BoutonVolume (Autodesk Fusion 360 design; units mm, degrees)
Autodesk Fusion 360 part; units mm, degrees
sketch "Revolution Sketch" plane through (0, 0, 0) normal (0, 1, 0) x (1, 0, 0)
  line L0 (5.5, 0) -> (0, 0)
  line L1 (5.6414, -11.9992) -> (5.5, 0)
  line L2 (-5.8686, 0) -> (0, 0) construction
  line L3 (5.6414, -12) -> (0, -12) construction
  arc A0 (0, -19) -> (12, -15.6532) centre (0.1354, 3.7013) ccw
  line L4 (11.9997, -11.2) -> (12, -13.3255) construction
  line L5 (12, -18.8) -> (12, -15.6532) construction
  line L6 (12, -14.6532) -> (12, -13.3255) construction
  line L7 (12, -18.8) -> (12, -15.6532) construction
  line L8 (12, -14.6532) -> (12, -13.3255) construction
  line L9 (0, -11.3) -> (11.9997, -11.2) construction
  arc A1 (12, -14.6532) -> (5.6414, -11.9992) centre (0.1775, -34.0336) ccw
  line L10 (5.6414, -12) -> (5.6414, -11.9992) construction
  line L11 (12, -15.6532) -> (12, -14.6532)
  line L12 (0, -19) -> (0, 0)
  line L13 (0, -19) -> (12, -19) construction
  point P0 (0, -6)
  dimension "d23" = 19
  dimension "d24" = 12
  dimension "d25" = 5.5
  dimension "d26" = 1
  dimension "d28" = 12
  constraint horizontal L0
  constraint horizontal L3
  constraint collinear L5 L6
  constraint collinear L7 L8
  constraint perpendicular L3 L10
  constraint perpendicular L2 L12
  constraint perpendicular L12 L13
  measures "d23" distance of L0.end A0.start
  measures "d24" distance of L0.start L1.start
  measures "d25" distance of L0.end L0.start
  measures "d26" vertical distance of A0.end L6.start
  measures "d28" distance of L11 L12
revolve "Revolve1" add sketch "Revolution Sketch" angle 360 about axis through (0, 0, 22.5431) along (0, 0, -1) makes body 1
sketch "Bottom" plane through (0, 0, 0) normal (0, 0, -1) x (1, 0, 0)
  circle A0 centre (0, 0) radius 5.5
  line L0 (2.5, -3) -> (-2.5, -3)
  line L1 (-2.5, -3) -> (-2.5, 3)
  line L2 (-2.5, 3) -> (2.5, 3)
  line L3 (2.5, 3) -> (2.5, -3)
  line L4 (2.5, -3) -> (-2.5, 3) construction
  line L5 (-2.5, -3) -> (2.5, 3) construction
  line L6 (0.98, 5.412) -> (0.98, 3)
  line L7 (0.98, 3) -> (-0.98, 3)
  line L8 (-0.98, 3) -> (-0.98, 5.412)
  line L9 (-1, -5.8) -> (1, -5.8) construction
  line L10 (1, -5.4083) -> (1, -3)
  line L11 (1, -3) -> (-1, -3)
  line L12 (-1, -3) -> (-1, -5.4083)
  line L13 (-0.98, 5.412) -> (-0.98, 5.8) construction
  line L14 (-0.98, 5.8) -> (0.98, 5.8) construction
  line L15 (0.98, 5.412) -> (0.98, 5.8) construction
  line L16 (-1, -5.4083) -> (-1, -5.8) construction
  line L17 (1, -5.4083) -> (1, -5.8) construction
  dimension "d7" = 5
  dimension "d8" = 6
  dimension "d10" = 2
  dimension "d12" = 2.8
  constraint horizontal L0
  constraint perpendicular L0 L1
  constraint parallel L0 L2
  constraint parallel L1 L3
  constraint coincident L4 A0.centre
  constraint coincident L5 A0.centre
  constraint coincident A0.centre origin
  constraint vertical L6
  constraint horizontal L7
  constraint vertical L8
  constraint horizontal L9
  constraint vertical L10
  constraint horizontal L11
  constraint vertical L12
  constraint coincident A0 L8.end
  constraint parallel L8 L13
  constraint coincident A0 L6.start
  constraint parallel L6 L15
  constraint coincident A0 L12.end
  constraint coincident A0 L10.start
  constraint perpendicular L9 L16
  constraint perpendicular L9 L17
  measures "d7" distance of L1.end L2.end
  measures "d8" distance of L0.end L1.end
  measures "d10" distance of L9.start L9.end
  measures "d12" distance of L9.end L10.end
extrude "Trou" cut sketch "Bottom" against normal blind 13 contours L0 L1 L2 L3 L7 L11 bodies 1
extrude "fente" cut sketch "Bottom" against normal blind 4 contours A0 L2 L6 L7 L8 | A0 L0 L10 L11 L12 bodies 1
ref_plane "WorkPlane1" through (0, 0, 14.65) normal (0, 0, 1) x (1, 0, 0)
sketch "Serrated circle" plane through (0, 0, 14.65) normal (0, 0, 1) x (1, 0, 0)
  line L0 (3, 3) -> (-3, 3)
  line L1 (-3, 3) -> (-3, -3)
  line L2 (-3, -3) -> (3, -3)
  line L3 (3, -3) -> (3, 3)
  circle A0 centre (0.0025, 0.0002) radius 12.5 construction
  line L4 (12.4997, 0.2655) -> (13.0382, -0.0013)
  line L5 (13.0382, -0.0013) -> (12.498, -0.3336)
  line L6 (12.4507, 1.1366) -> (13.0066, 0.908)
  line L7 (13.0066, 0.908) -> (12.4909, 0.5389)
  line L8 (12.3411, 2.0022) -> (12.9116, 1.8129)
  line L9 (12.9116, 1.8129) -> (12.4229, 1.4087)
  line L10 (12.1714, 2.858) -> (12.7537, 2.709)
  line L11 (12.7537, 2.709) -> (12.2944, 2.2717)
  line L12 (11.9424, 3.6999) -> (12.5336, 3.5919)
  line L13 (12.5336, 3.5919) -> (12.106, 3.1236)
  line L14 (11.6553, 4.5238) -> (12.2526, 4.4573)
  line L15 (12.2526, 4.4573) -> (11.8586, 3.9603)
  line L16 (11.3113, 5.3256) -> (11.9118, 5.3009)
  line L17 (11.9118, 5.3009) -> (11.5535, 4.7777)
  line L18 (10.9123, 6.1015) -> (11.5131, 6.1188)
  line L19 (11.5131, 6.1188) -> (11.1921, 5.5718)
  line L20 (10.4601, 6.8477) -> (11.0582, 6.9068)
  line L21 (11.0582, 6.9068) -> (10.7762, 6.3388)
  line L22 (9.957, 7.5605) -> (10.5495, 7.6612)
  line L23 (10.5495, 7.6612) -> (10.3078, 7.0749)
  line L24 (9.4054, 8.2365) -> (9.9894, 8.3782)
  line L25 (9.9894, 8.3782) -> (9.7892, 7.7765)
  line L26 (8.8079, 8.8723) -> (9.3807, 9.0545)
  line L27 (9.3807, 9.0545) -> (9.2229, 8.4402)
  line L28 (8.1676, 9.465) -> (8.7262, 9.6866)
  line L29 (8.7262, 9.6866) -> (8.6117, 9.0629)
  line L30 (7.4875, 10.0115) -> (8.0293, 10.2716)
  line L31 (8.0293, 10.2716) -> (7.9586, 9.6413)
  line L32 (6.7709, 10.5092) -> (7.2932, 10.8065)
  line L33 (7.2932, 10.8065) -> (7.2666, 10.1728)
  line L34 (6.0213, 10.9557) -> (6.5217, 11.2887)
  line L35 (6.5217, 11.2887) -> (6.5393, 10.6548)
  line L36 (5.2425, 11.3489) -> (5.7183, 11.716)
  line L37 (5.7183, 11.716) -> (5.7802, 11.0848)
  line L38 (4.4381, 11.6868) -> (4.8872, 12.0861)
  line L39 (4.8872, 12.0861) -> (4.9929, 11.4608)
  line L40 (3.612, 11.9677) -> (4.0322, 12.3974)
  line L41 (4.0322, 12.3974) -> (4.1813, 11.781)
  line L42 (2.7684, 12.1904) -> (3.1576, 12.6483)
  line L43 (3.1576, 12.6483) -> (3.3493, 12.0438)
  line L44 (1.9114, 12.3536) -> (2.2676, 12.8376)
  line L45 (2.2676, 12.8376) -> (2.5011, 12.248)
  line L46 (1.045, 12.4567) -> (1.3666, 12.9644)
  line L47 (1.3666, 12.9644) -> (1.6406, 12.3924)
  line L48 (0.1735, 12.4991) -> (0.459, 13.0279)
  line L49 (0.459, 13.0279) -> (0.7722, 12.4765)
  line L50 (-0.6988, 12.4805) -> (-0.4509, 13.028)
  line L51 (-0.4509, 13.028) -> (-0.1, 12.4998)
  line L52 (-1.5676, 12.4012) -> (-1.3586, 12.9647)
  line L53 (-1.3586, 12.9647) -> (-0.9717, 12.4622)
  line L54 (-2.4289, 12.2615) -> (-2.2596, 12.8381)
  line L55 (-2.2596, 12.8381) -> (-1.8386, 12.3639)
  line L56 (-3.2783, 12.062) -> (-3.1496, 12.6491)
  line L57 (-3.1496, 12.6491) -> (-2.6966, 12.2053)
  line L58 (-4.1116, 11.8038) -> (-4.0243, 12.3984)
  line L59 (-4.0243, 12.3984) -> (-3.5414, 11.9873)
  line L60 (-4.925, 11.488) -> (-4.8793, 12.0873)
  line L61 (-4.8793, 12.0873) -> (-4.3689, 11.7109)
  line L62 (-5.7143, 11.1163) -> (-5.7106, 11.7173)
  line L63 (-5.7106, 11.7173) -> (-5.1752, 11.3775)
  line L64 (-6.4758, 10.6905) -> (-6.514, 11.2902)
  line L65 (-6.514, 11.2902) -> (-5.9562, 10.9886)
  line L66 (-7.2058, 10.2125) -> (-7.2857, 10.8082)
  line L67 (-7.2857, 10.8082) -> (-6.7082, 10.5461)
  line L68 (-7.9006, 9.6848) -> (-8.0219, 10.2734)
  line L69 (-8.0219, 10.2734) -> (-7.4275, 10.0523)
  line L70 (-8.5569, 9.1099) -> (-8.719, 9.6887)
  line L71 (-8.719, 9.6887) -> (-8.1106, 9.5096)
  line L72 (-9.1715, 8.4907) -> (-9.3735, 9.0567)
  line L73 (-9.3735, 9.0567) -> (-8.7542, 8.9205)
  line L74 (-9.7414, 7.83) -> (-9.9824, 8.3806)
  line L75 (-9.9824, 8.3806) -> (-9.3551, 8.2879)
  line L76 (-10.2639, 7.1313) -> (-10.5427, 7.6636)
  line L77 (-10.5427, 7.6636) -> (-9.9104, 7.615)
  line L78 (-10.7363, 6.3977) -> (-11.0516, 6.9094)
  line L79 (-11.0516, 6.9094) -> (-10.4174, 6.9049)
  line L80 (-11.1564, 5.6331) -> (-11.5066, 6.1215)
  line L81 (-11.5066, 6.1215) -> (-10.8737, 6.1612)
  line L82 (-11.5221, 4.8409) -> (-11.9056, 5.3037)
  line L83 (-11.9056, 5.3037) -> (-11.277, 5.3875)
  line L84 (-11.8317, 4.0252) -> (-12.2465, 4.4601)
  line L85 (-12.2465, 4.4601) -> (-11.6253, 4.5876)
  line L86 (-12.0837, 3.1899) -> (-12.5278, 3.5948)
  line L87 (-12.5278, 3.5948) -> (-11.917, 3.7653)
  line L88 (-12.2767, 2.339) -> (-12.748, 2.712)
  line L89 (-12.748, 2.712) -> (-12.1506, 2.9247)
  line L90 (-12.41, 1.4768) -> (-12.9061, 1.8159)
  line L91 (-12.9061, 1.8159) -> (-12.325, 2.0698)
  line L92 (-12.4827, 0.6073) -> (-13.0013, 0.9111)
  line L93 (-13.0013, 0.9111) -> (-12.4393, 1.2048)
  line L94 (-12.4947, -0.2651) -> (-13.0332, 0.0017)
  line L95 (-13.0332, 0.0017) -> (-12.493, 0.334)
  line L96 (-12.4457, -1.1362) -> (-13.0016, -0.9076)
  line L97 (-13.0016, -0.9076) -> (-12.4859, -0.5384)
  line L98 (-12.3361, -2.0018) -> (-12.9065, -1.8125)
  line L99 (-12.9065, -1.8125) -> (-12.4179, -1.4083)
  line L100 (-12.1664, -2.8576) -> (-12.7487, -2.7086)
  line L101 (-12.7487, -2.7086) -> (-12.2894, -2.2713)
  line L102 (-11.9374, -3.6995) -> (-12.5286, -3.5914)
  line L103 (-12.5286, -3.5914) -> (-12.101, -3.1232)
  line L104 (-11.6503, -4.5234) -> (-12.2476, -4.4568)
  line L105 (-12.2476, -4.4568) -> (-11.8536, -3.9598)
  line L106 (-11.3063, -5.3252) -> (-11.9068, -5.3005)
  line L107 (-11.9068, -5.3005) -> (-11.5485, -4.7772)
  line L108 (-10.9073, -6.1011) -> (-11.5081, -6.1183)
  line L109 (-11.5081, -6.1183) -> (-11.1871, -5.5714)
  line L110 (-10.4551, -6.8473) -> (-11.0532, -6.9064)
  line L111 (-11.0532, -6.9064) -> (-10.7712, -6.3383)
  line L112 (-9.952, -7.5601) -> (-10.5445, -7.6607)
  line L113 (-10.5445, -7.6607) -> (-10.3028, -7.0744)
  line L114 (-9.4004, -8.236) -> (-9.9844, -8.3778)
  line L115 (-9.9844, -8.3778) -> (-9.7842, -7.7761)
  line L116 (-8.8029, -8.8719) -> (-9.3757, -9.054)
  line L117 (-9.3757, -9.054) -> (-9.2179, -8.4398)
  line L118 (-8.1626, -9.4645) -> (-8.7212, -9.6862)
  line L119 (-8.7212, -9.6862) -> (-8.6067, -9.0624)
  line L120 (-7.4825, -10.011) -> (-8.0243, -10.2711)
  line L121 (-8.0243, -10.2711) -> (-7.9535, -9.6409)
  line L122 (-6.7659, -10.5088) -> (-7.2882, -10.806)
  line L123 (-7.2882, -10.806) -> (-7.2616, -10.1724)
  line L124 (-6.0163, -10.9553) -> (-6.5167, -11.2883)
  line L125 (-6.5167, -11.2883) -> (-6.5343, -10.6543)
  line L126 (-5.2375, -11.3485) -> (-5.7133, -11.7155)
  line L127 (-5.7133, -11.7155) -> (-5.7752, -11.0844)
  line L128 (-4.433, -11.6863) -> (-4.8822, -12.0857)
  line L129 (-4.8822, -12.0857) -> (-4.9879, -11.4604)
  line L130 (-3.607, -11.9673) -> (-4.0272, -12.397)
  line L131 (-4.0272, -12.397) -> (-4.1763, -11.7806)
  line L132 (-2.7634, -12.1899) -> (-3.1526, -12.6479)
  line L133 (-3.1526, -12.6479) -> (-3.3443, -12.0434)
  line L134 (-1.9063, -12.3532) -> (-2.2626, -12.8372)
  line L135 (-2.2626, -12.8372) -> (-2.496, -12.2475)
  line L136 (-1.04, -12.4562) -> (-1.3616, -12.9639)
  line L137 (-1.3616, -12.9639) -> (-1.6356, -12.392)
  line L138 (-0.1685, -12.4986) -> (-0.454, -13.0275)
  line L139 (-0.454, -13.0275) -> (-0.7672, -12.4761)
  line L140 (0.7038, -12.4801) -> (0.4559, -13.0276)
  line L141 (0.4559, -13.0276) -> (0.105, -12.4994)
  line L142 (1.5727, -12.4008) -> (1.3636, -12.9642)
  line L143 (1.3636, -12.9642) -> (0.9767, -12.4618)
  line L144 (2.4339, -12.261) -> (2.2646, -12.8377)
  line L145 (2.2646, -12.8377) -> (1.8436, -12.3634)
  line L146 (3.2833, -12.0616) -> (3.1546, -12.6486)
  line L147 (3.1546, -12.6486) -> (2.7016, -12.2049)
  line L148 (4.1167, -11.8033) -> (4.0293, -12.3979)
  line L149 (4.0293, -12.3979) -> (3.5464, -11.9869)
  line L150 (4.93, -11.4876) -> (4.8844, -12.0868)
  line L151 (4.8844, -12.0868) -> (4.3739, -11.7105)
  line L152 (5.7194, -11.1159) -> (5.7156, -11.7169)
  line L153 (5.7156, -11.7169) -> (5.1802, -11.377)
  line L154 (6.4808, -10.69) -> (6.519, -11.2898)
  line L155 (6.519, -11.2898) -> (5.9612, -10.9881)
  line L156 (7.2108, -10.2121) -> (7.2907, -10.8077)
  line L157 (7.2907, -10.8077) -> (6.7132, -10.5457)
  line L158 (7.9056, -9.6844) -> (8.0269, -10.273)
  line L159 (8.0269, -10.273) -> (7.4325, -10.0519)
  line L160 (8.5619, -9.1095) -> (8.724, -9.6882)
  line L161 (8.724, -9.6882) -> (8.1156, -9.5091)
  line L162 (9.1765, -8.4902) -> (9.3785, -9.0562)
  line L163 (9.3785, -9.0562) -> (8.7592, -8.92)
  line L164 (9.7464, -7.8296) -> (9.9875, -8.3801)
  line L165 (9.9875, -8.3801) -> (9.3601, -8.2875)
  line L166 (10.2689, -7.1308) -> (10.5477, -7.6632)
  line L167 (10.5477, -7.6632) -> (9.9154, -7.6145)
  line L168 (10.7413, -6.3973) -> (11.0566, -6.9089)
  line L169 (11.0566, -6.9089) -> (10.4224, -6.9045)
  line L170 (11.1614, -5.6326) -> (11.5116, -6.121)
  line L171 (11.5116, -6.121) -> (10.8787, -6.1608)
  line L172 (11.5272, -4.8405) -> (11.9106, -5.3033)
  line L173 (11.9106, -5.3033) -> (11.282, -5.3871)
  line L174 (11.8368, -4.0248) -> (12.2515, -4.4597)
  line L175 (12.2515, -4.4597) -> (11.6303, -4.5872)
  line L176 (12.0887, -3.1895) -> (12.5328, -3.5944)
  line L177 (12.5328, -3.5944) -> (11.922, -3.7649)
  line L178 (12.2818, -2.3386) -> (12.753, -2.7115)
  line L179 (12.753, -2.7115) -> (12.1556, -2.9242)
  line L180 (12.415, -1.4763) -> (12.9111, -1.8155)
  line L181 (12.9111, -1.8155) -> (12.33, -2.0694)
  line L182 (12.4878, -0.6069) -> (13.0063, -0.9106)
  line L183 (13.0063, -0.9106) -> (12.4443, -1.2044)
  line L184 (12.4997, 0.2655) -> (12.4909, 0.5389)
  line L185 (12.4507, 1.1366) -> (12.4229, 1.4087)
  line L186 (12.3411, 2.0022) -> (12.2944, 2.2717)
  line L187 (12.1714, 2.858) -> (12.106, 3.1236)
  line L188 (11.9424, 3.6999) -> (11.8586, 3.9603)
  line L189 (11.6553, 4.5238) -> (11.5535, 4.7777)
  line L190 (11.3113, 5.3256) -> (11.1921, 5.5718)
  line L191 (10.9123, 6.1015) -> (10.7762, 6.3388)
  line L192 (10.4601, 6.8477) -> (10.3078, 7.0749)
  line L193 (9.957, 7.5605) -> (9.7892, 7.7765)
  line L194 (9.4054, 8.2365) -> (9.2229, 8.4402)
  line L195 (8.8079, 8.8723) -> (8.6117, 9.0629)
  line L196 (8.1676, 9.465) -> (7.9586, 9.6413)
  line L197 (7.4875, 10.0115) -> (7.2666, 10.1728)
  line L198 (6.7709, 10.5092) -> (6.5393, 10.6548)
  line L199 (6.0213, 10.9557) -> (5.7802, 11.0848)
  line L200 (5.2425, 11.3489) -> (4.9929, 11.4608)
  line L201 (4.4381, 11.6868) -> (4.1813, 11.781)
  line L202 (3.612, 11.9677) -> (3.3493, 12.0438)
  line L203 (2.7684, 12.1904) -> (2.5011, 12.248)
  line L204 (1.9114, 12.3536) -> (1.6406, 12.3924)
  line L205 (1.045, 12.4567) -> (0.7722, 12.4765)
  line L206 (0.1735, 12.4991) -> (-0.1, 12.4998)
  line L207 (-0.6988, 12.4805) -> (-0.9717, 12.4622)
  line L208 (-1.5676, 12.4012) -> (-1.8386, 12.3639)
  line L209 (-2.4289, 12.2615) -> (-2.6966, 12.2053)
  line L210 (-3.2783, 12.062) -> (-3.5414, 11.9873)
  line L211 (-4.1116, 11.8038) -> (-4.3689, 11.7109)
  line L212 (-4.925, 11.488) -> (-5.1752, 11.3775)
  line L213 (-5.7143, 11.1163) -> (-5.9562, 10.9886)
  line L214 (-6.4758, 10.6905) -> (-6.7082, 10.5461)
  line L215 (-7.2058, 10.2125) -> (-7.4275, 10.0523)
  line L216 (-7.9006, 9.6848) -> (-8.1106, 9.5096)
  line L217 (-8.5569, 9.1099) -> (-8.7542, 8.9205)
  line L218 (-9.1715, 8.4907) -> (-9.3551, 8.2879)
  line L219 (-9.7414, 7.83) -> (-9.9104, 7.615)
  line L220 (-10.2639, 7.1313) -> (-10.4174, 6.9049)
  line L221 (-10.7363, 6.3977) -> (-10.8737, 6.1612)
  line L222 (-11.1564, 5.6331) -> (-11.277, 5.3875)
  line L223 (-11.5221, 4.8409) -> (-11.6253, 4.5876)
  line L224 (-11.8317, 4.0252) -> (-11.917, 3.7653)
  line L225 (-12.0837, 3.1899) -> (-12.1506, 2.9247)
  line L226 (-12.2767, 2.339) -> (-12.325, 2.0698)
  line L227 (-12.41, 1.4768) -> (-12.4393, 1.2048)
  line L228 (-12.4827, 0.6073) -> (-12.493, 0.334)
  line L229 (-12.4947, -0.2651) -> (-12.4859, -0.5384)
  line L230 (-12.4457, -1.1362) -> (-12.4179, -1.4083)
  line L231 (-12.3361, -2.0018) -> (-12.2894, -2.2713)
  line L232 (-12.1664, -2.8576) -> (-12.101, -3.1232)
  line L233 (-11.9374, -3.6995) -> (-11.8536, -3.9598)
  line L234 (-11.6503, -4.5234) -> (-11.5485, -4.7772)
  line L235 (-11.3063, -5.3252) -> (-11.1871, -5.5714)
  line L236 (-10.9073, -6.1011) -> (-10.7712, -6.3383)
  line L237 (-10.4551, -6.8473) -> (-10.3028, -7.0744)
  line L238 (-9.952, -7.5601) -> (-9.7842, -7.7761)
  line L239 (-9.4004, -8.236) -> (-9.2179, -8.4398)
  line L240 (-8.8029, -8.8719) -> (-8.6067, -9.0624)
  line L241 (-8.1626, -9.4645) -> (-7.9535, -9.6409)
  line L242 (-7.4825, -10.011) -> (-7.2616, -10.1724)
  line L243 (-6.7659, -10.5088) -> (-6.5343, -10.6543)
  line L244 (-6.0163, -10.9553) -> (-5.7752, -11.0844)
  line L245 (-5.2375, -11.3485) -> (-4.9879, -11.4604)
  line L246 (-4.433, -11.6863) -> (-4.1763, -11.7806)
  line L247 (-3.607, -11.9673) -> (-3.3443, -12.0434)
  line L248 (-2.7634, -12.1899) -> (-2.496, -12.2475)
  line L249 (-1.9063, -12.3532) -> (-1.6356, -12.392)
  line L250 (-1.04, -12.4562) -> (-0.7672, -12.4761)
  line L251 (-0.1685, -12.4986) -> (0.105, -12.4994)
  line L252 (0.7038, -12.4801) -> (0.9767, -12.4618)
  line L253 (1.5727, -12.4008) -> (1.8436, -12.3634)
  line L254 (2.4339, -12.261) -> (2.7016, -12.2049)
  line L255 (3.2833, -12.0616) -> (3.5464, -11.9869)
  line L256 (4.1167, -11.8033) -> (4.3739, -11.7105)
  line L257 (4.93, -11.4876) -> (5.1802, -11.377)
  line L258 (5.7194, -11.1159) -> (5.9612, -10.9881)
  line L259 (6.4808, -10.69) -> (6.7132, -10.5457)
  line L260 (7.2108, -10.2121) -> (7.4325, -10.0519)
  line L261 (7.9056, -9.6844) -> (8.1156, -9.5091)
  line L262 (8.5619, -9.1095) -> (8.7592, -8.92)
  line L263 (9.1765, -8.4902) -> (9.3601, -8.2875)
  line L264 (9.7464, -7.8296) -> (9.9154, -7.6145)
  line L265 (10.2689, -7.1308) -> (10.4224, -6.9045)
  line L266 (10.7413, -6.3973) -> (10.8787, -6.1608)
  line L267 (11.1614, -5.6326) -> (11.282, -5.3871)
  line L268 (11.5272, -4.8405) -> (11.6303, -4.5872)
  line L269 (11.8368, -4.0248) -> (11.922, -3.7649)
  line L270 (12.0887, -3.1895) -> (12.1556, -2.9242)
  line L271 (12.2818, -2.3386) -> (12.33, -2.0694)
  line L272 (12.415, -1.4763) -> (12.4443, -1.2044)
  line L273 (12.4878, -0.6069) -> (12.498, -0.3336)
  dimension "d18" = 360
  dimension "d29" = 25
  constraint coincident A0 L5.end
  constraint coincident A0 L4.start
  measures "d29" diameter of A0
extrude "dentelure" add sketch "Serrated circle" along normal blind 1 separate body makes body 2
